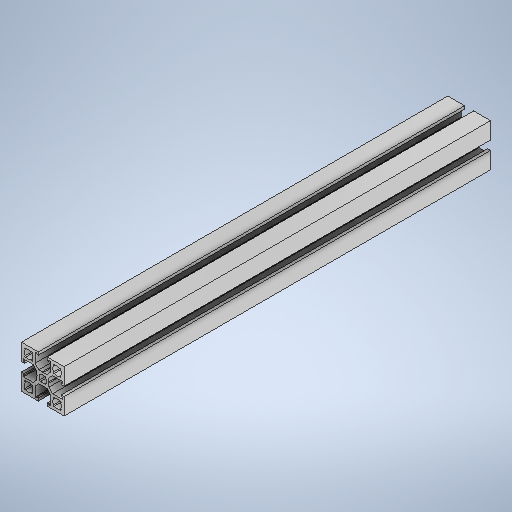
# Autodesk Inventor part: 3030 Aluminium Profile
Saved by Autodesk Inventor 2026.2 (Build 302298010, 298A)
## iProperties
Created: 2022-09-09
Part Number: 3030 Aluminium Profile
Material: Aluminum 6061-AHC
Document SubType Name: Modeling
Designer: chanh
Density: 2.7 g/cm^3
Appearance: Aluminum - Dark
Author: chanh
Autodesk Inventor part; units mm, degrees
ref_plane "RIGHT" through (0, 0, 0) normal (1, 0, 0) x (0, 1, 0)
ref_plane "TOP" through (0, 0, 0) normal (0, 1, 0) x (-1, 0, 0)
ref_plane "FRONT" through (0, 0, 0) normal (0, 0, 1) x (1, 0, 0)
sketch "Sketch2" plane through (0, 0, 0) normal (0, 0, 1) x (1, 0, 0)
  circle A0 centre (0, 0) radius 2.5
  circle A1 centre (10, 10) radius 3
  line L0 (-4.25, -4.25) -> (4.25, -4.25)
  line L1 (4.25, -4.25) -> (4.25, 4.25)
  line L2 (4.25, 4.25) -> (-4.25, 4.25)
  line L3 (-4.25, 4.25) -> (-4.25, -4.25)
  line L4 (-4.25, -4.25) -> (4.25, 4.25) construction
  line L5 (4.25, -4.25) -> (-4.25, 4.25) construction
  line L6 (15, 5) -> (15, 15)
  line L7 (15, 15) -> (5, 15)
  line L8 (5, 5) -> (15, 15) construction
  line L9 (15, 5) -> (5, 15) construction
  line L10 (5, 15) -> (3.15, 15)
  line L11 (3.15, 15) -> (3.15, 13)
  line L12 (3.15, 13) -> (4.15, 13)
  line L13 (4.15, 13) -> (4.15, 13.7)
  line L14 (4.15, 13.7) -> (5.5, 13.7)
  line L15 (0, 0) -> (10, 10) construction
  line L16 (5.5, 15) -> (5.5, 5.5)
  line L17 (5.5, 5.5) -> (15, 5.5)
  line L18 (2.8358, 4.25) -> (5.5, 6.9142)
  line L19 (12.4042, 7.5958) -> (7.5958, 12.4042) construction
  line L20 (12.1213, 7.313) -> (7.313, 12.1213)
  line L21 (7.8787, 12.687) -> (12.687, 7.8787)
  arc A2 (12.1213, 7.313) -> (12.687, 7.8787) centre (12.4042, 7.5958) ccw
  arc A3 (7.8787, 12.687) -> (7.313, 12.1213) centre (7.5958, 12.4042) ccw
  line L22 (-0.4, 4.25) -> (0, 3.85)
  line L23 (0, 3.85) -> (0.4, 4.25)
  line L24 (0, 4.25) -> (0, -4.25) construction
  line L25 (7.5958, 7.5958) -> (12.4042, 12.4042) construction
  line L26 (7.8787, 7.313) -> (12.687, 12.1213)
  line L27 (12.1213, 12.687) -> (7.313, 7.8787)
  arc A4 (7.313, 7.8787) -> (7.8787, 7.313) centre (7.5958, 7.5958) ccw
  arc A5 (12.687, 12.1213) -> (12.1213, 12.687) centre (12.4042, 12.4042) ccw
  line L28 (15, 5) -> (15, 3.15)
  line L29 (15, 3.15) -> (13, 3.15)
  line L30 (13, 3.15) -> (13, 4.15)
  line L31 (13, 4.15) -> (13.7, 4.15)
  line L32 (13.7, 4.15) -> (13.7, 5.5)
  line L33 (4.25, 2.8358) -> (6.9142, 5.5)
  line L34 (-1.7678, -1.7678) -> (1.7678, 1.7678) construction
  line L35 (-1.4142, -2.1213) -> (2.1213, 1.4142)
  line L36 (1.4142, 2.1213) -> (-2.1213, -1.4142)
  arc A6 (-2.1213, -1.4142) -> (-1.4142, -2.1213) centre (-1.7678, -1.7678) ccw
  arc A7 (2.1213, 1.4142) -> (1.4142, 2.1213) centre (1.7678, 1.7678) ccw
  line L37 (1.7678, -1.7678) -> (-1.7678, 1.7678) construction
  line L38 (2.1213, -1.4142) -> (-1.4142, 2.1213)
  line L39 (-2.1213, 1.4142) -> (1.4142, -2.1213)
  arc A8 (1.4142, -2.1213) -> (2.1213, -1.4142) centre (1.7678, -1.7678) ccw
  arc A9 (-1.4142, 2.1213) -> (-2.1213, 1.4142) centre (-1.7678, 1.7678) ccw
  line L40 (-4.25, 0) -> (4.25, 0) construction
  circle A10 centre (10, -10) radius 3
  line L41 (15, -5) -> (15, -15)
  line L42 (15, -15) -> (5, -15)
  line L43 (5, -5) -> (15, -15) construction
  line L44 (15, -5) -> (5, -15) construction
  line L45 (5, -15) -> (3.15, -15)
  line L46 (3.15, -15) -> (3.15, -13)
  line L47 (3.15, -13) -> (4.15, -13)
  line L48 (4.15, -13) -> (4.15, -13.7)
  line L49 (4.15, -13.7) -> (5.5, -13.7)
  line L50 (0, 0) -> (10, -10) construction
  line L51 (5.5, -15) -> (5.5, -5.5)
  line L52 (5.5, -5.5) -> (15, -5.5)
  line L53 (2.8358, -4.25) -> (5.5, -6.9142)
  line L54 (12.4042, -7.5958) -> (7.5958, -12.4042) construction
  line L55 (12.1213, -7.313) -> (7.313, -12.1213)
  line L56 (7.8787, -12.687) -> (12.687, -7.8787)
  arc A11 (12.687, -7.8787) -> (12.1213, -7.313) centre (12.4042, -7.5958) ccw
  arc A12 (7.313, -12.1213) -> (7.8787, -12.687) centre (7.5958, -12.4042) ccw
  line L57 (7.5958, -7.5958) -> (12.4042, -12.4042) construction
  line L58 (7.8787, -7.313) -> (12.687, -12.1213)
  line L59 (12.1213, -12.687) -> (7.313, -7.8787)
  arc A13 (7.8787, -7.313) -> (7.313, -7.8787) centre (7.5958, -7.5958) ccw
  arc A14 (12.1213, -12.687) -> (12.687, -12.1213) centre (12.4042, -12.4042) ccw
  line L60 (13.7, -4.15) -> (13.7, -5.5)
  line L61 (15, -5) -> (15, -3.15)
  line L62 (15, -3.15) -> (13, -3.15)
  line L63 (13, -4.15) -> (13.7, -4.15)
  line L64 (13, -3.15) -> (13, -4.15)
  line L65 (4.25, -2.8358) -> (6.9142, -5.5)
  circle A15 centre (-10, 10) radius 3
  line L66 (-15, 5) -> (-15, 15)
  line L67 (-15, 15) -> (-5, 15)
  line L68 (-5, 5) -> (-15, 15) construction
  line L69 (-15, 5) -> (-5, 15) construction
  line L70 (-5, 15) -> (-3.15, 15)
  line L71 (-3.15, 15) -> (-3.15, 13)
  line L72 (-3.15, 13) -> (-4.15, 13)
  line L73 (-4.15, 13) -> (-4.15, 13.7)
  line L74 (-4.15, 13.7) -> (-5.5, 13.7)
  line L75 (0, 0) -> (-10, 10) construction
  line L76 (-5.5, 15) -> (-5.5, 5.5)
  line L77 (-5.5, 5.5) -> (-15, 5.5)
  line L78 (-2.8358, 4.25) -> (-5.5, 6.9142)
  line L79 (-12.4042, 7.5958) -> (-7.5958, 12.4042) construction
  line L80 (-12.1213, 7.313) -> (-7.313, 12.1213)
  line L81 (-7.8787, 12.687) -> (-12.687, 7.8787)
  arc A16 (-12.687, 7.8787) -> (-12.1213, 7.313) centre (-12.4042, 7.5958) ccw
  arc A17 (-7.313, 12.1213) -> (-7.8787, 12.687) centre (-7.5958, 12.4042) ccw
  line L82 (-7.5958, 7.5958) -> (-12.4042, 12.4042) construction
  line L83 (-7.8787, 7.313) -> (-12.687, 12.1213)
  line L84 (-12.1213, 12.687) -> (-7.313, 7.8787)
  arc A18 (-7.8787, 7.313) -> (-7.313, 7.8787) centre (-7.5958, 7.5958) ccw
  arc A19 (-12.1213, 12.687) -> (-12.687, 12.1213) centre (-12.4042, 12.4042) ccw
  line L85 (-13.7, 4.15) -> (-13.7, 5.5)
  line L86 (-15, 5) -> (-15, 3.15)
  line L87 (-15, 3.15) -> (-13, 3.15)
  line L88 (-13, 4.15) -> (-13.7, 4.15)
  line L89 (-13, 3.15) -> (-13, 4.15)
  line L90 (-4.25, 2.8358) -> (-6.9142, 5.5)
  arc A20 (-12.687, -12.1213) -> (-12.1213, -12.687) centre (-12.4042, -12.4042) ccw
  arc A21 (-7.8787, -12.687) -> (-7.313, -12.1213) centre (-7.5958, -12.4042) ccw
  arc A22 (-12.1213, -7.313) -> (-12.687, -7.8787) centre (-12.4042, -7.5958) ccw
  line L91 (-12.1213, -12.687) -> (-7.313, -7.8787)
  line L92 (-7.8787, -12.687) -> (-12.687, -7.8787)
  line L93 (-7.5958, -7.5958) -> (-12.4042, -12.4042) construction
  line L94 (-12.4042, -7.5958) -> (-7.5958, -12.4042) construction
  line L95 (-7.8787, -7.313) -> (-12.687, -12.1213)
  line L96 (-12.1213, -7.313) -> (-7.313, -12.1213)
  circle A23 centre (-10, -10) radius 3
  line L97 (-15, -15) -> (-5, -15)
  line L98 (-15, -5) -> (-15, -15)
  line L99 (-5.5, -15) -> (-5.5, -5.5)
  line L100 (-5.5, -5.5) -> (-15, -5.5)
  line L101 (-15, -5) -> (-5, -15) construction
  line L102 (-5, -5) -> (-15, -15) construction
  arc A24 (-7.313, -7.8787) -> (-7.8787, -7.313) centre (-7.5958, -7.5958) ccw
  line L103 (-5, -15) -> (-3.15, -15)
  line L104 (-3.15, -15) -> (-3.15, -13)
  line L105 (-4.15, -13) -> (-4.15, -13.7)
  line L106 (-4.15, -13.7) -> (-5.5, -13.7)
  line L107 (-3.15, -13) -> (-4.15, -13)
  line L108 (0, 0) -> (-10, -10) construction
  line L109 (-2.8358, -4.25) -> (-5.5, -6.9142)
  line L110 (-4.25, -2.8358) -> (-6.9142, -5.5)
  line L111 (-13.7, -4.15) -> (-13.7, -5.5)
  line L112 (-15, -5) -> (-15, -3.15)
  line L113 (-13, -3.15) -> (-13, -4.15)
  line L114 (-15, -3.15) -> (-13, -3.15)
  line L115 (-13, -4.15) -> (-13.7, -4.15)
  line L116 (-3.85, 0) -> (-4.25, 0.4)
  line L117 (-4.25, -0.4) -> (-3.85, 0)
  line L118 (0, -3.85) -> (-0.4, -4.25)
  line L119 (0.4, -4.25) -> (0, -3.85)
  line L120 (3.85, 0) -> (4.25, -0.4)
  line L121 (4.25, 0.4) -> (3.85, 0)
  point P0 (-7.6148, -8.1805)
  point P1 (-7.6148, -11.8195)
  point P2 (-8.1805, -12.3852)
  point P3 (-11.8195, -12.3852)
  point P4 (-12.3852, -11.8195)
  point P5 (-12.3852, -8.1805)
  point P6 (-11.8195, -7.6148)
  point P7 (-8.1805, -7.6148)
  point P8 (-7.6148, 11.8195)
  point P9 (-7.6148, 8.1805)
  point P10 (-8.1805, 7.6148)
  point P11 (-11.8195, 7.6148)
  point P12 (-12.3852, 8.1805)
  point P13 (-12.3852, 11.8195)
  point P14 (-11.8195, 12.3852)
  point P15 (-8.1805, 12.3852)
  point P16 (11.8195, -12.3852)
  point P17 (8.1805, -12.3852)
  point P18 (7.6148, -11.8195)
  point P19 (7.6148, -8.1805)
  point P20 (8.1805, -7.6148)
  point P21 (11.8195, -7.6148)
  point P22 (12.3852, -8.1805)
  point P23 (12.3852, -11.8195)
  point P24 (-2.0856, -1.3785)
  point P25 (-2.0856, 1.3785)
  point P26 (-1.3785, 2.0856)
  point P27 (1.3785, 2.0856)
  point P28 (2.0856, 1.3785)
  point P29 (2.0856, -1.3785)
  point P30 (1.3785, -2.0856)
  point P31 (-1.3785, -2.0856)
  point P32 (11.8195, 7.6148)
  point P33 (8.1805, 7.6148)
  point P34 (7.6148, 8.1805)
  point P35 (7.6148, 11.8195)
  point P36 (8.1805, 12.3852)
  point P37 (11.8195, 12.3852)
  point P38 (12.3852, 11.8195)
  point P39 (12.3852, 8.1805)
  dimension "d15" = 5
  dimension "d16" = 6
  dimension "d17" = 10
  dimension "d18" = 10
  dimension "d19" = 8.5
  dimension "d21" = 3.15
  dimension "d22" = 1
  dimension "d23" = 2
  dimension "d24" = 1.3
  dimension "d25" = 5
  dimension "d26" = 4.5
  dimension "d27" = 1
  dimension "d28" = 0.8
  dimension "d29" = 3.4
  dimension "d30" = 0.8
  dimension "d31" = 0.8
  dimension "d32" = 3.4
  dimension "d33" = 1
  dimension "d34" = 1
  dimension "d37" = 360
  constraints: 264 end point, 112 symmetric about line, 42 point on circle, 38 point on line, 25 centre point, 16 midpoint, 16 tangent, 10 perpendicular, 7 parallel, 2 horizontal, 1 coincident, 1 collinear, 1 vertical, 36 other
  measures "d15" diameter of A0
  measures "d16" diameter of A1
  measures "d17" horizontal distance of L15.end point (0, 0)
  measures "d18" horizontal distance of L15.end point (0, 0)
  measures "d19" distance of L2.end L1.end
  measures "d21" distance from line of L11 point (0, 0)
  measures "d22" distance between parallel lines of L13 L11
  measures "d23" distance between parallel lines of L12 L10
  measures "d24" distance between parallel lines of L10 L14
  measures "d25" horizontal distance of L6.end L15.end
  measures "d26" distance from line of L15.end L16
  measures "d27" distance between parallel lines of L8 L18
  measures "d28" distance between parallel lines of L21 L20
  measures "d29" distance of L15.end L19.end
  measures "d30" distance of L23.end L22.start
  measures "d31" diameter of A5
  measures "d32" distance of L25.end L15.end
  measures "d33" diameter of A7
  measures "d34" diameter of A9
extrude "Extrusion2" add sketch "Sketch2" along normal blind 300 contours L3 L117 L116 L2 L22 L23 L1 L121 L120 L0 L119 L118 | L0 L109 L99 L100 L110 L3 | L99 L97 L98 L100 | L106 L105 L107 L104 L103 L97 L99 | L100 L98 L112 L114 L113 L115 L111 | L0 L1 L65 L52 L51 L53 | L90 L77 L76 L78 L2 L3 | L51 L52 L41 L42 | L77 L66 L67 L76 | L51 L42 L45 L46 L47 L48 L49 | L85 L88 L89 L87 L86 L66 L77 | L60 L63 L64 L62 L61 L41 L52 | L76 L67 L70 L71 L72 L73 L74 | L1 L2 L18 L16 L17 L33 | L17 L16 L7 L6 | L17 L6 L28 L29 L30 L31 L32 | L14 L13 L12 L11 L10 L7 L16
body "Solid2"
